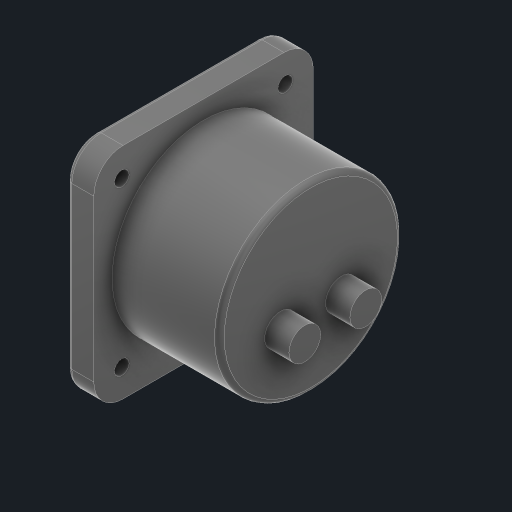
# Autodesk Inventor part: IIImeter
Saved by Autodesk Inventor 2024 (Build 280153000, 153)
## iProperties
Created: 2023-12-09
Part Number: IIImeter
Material: Acetal Resin, Black
Document SubType Name: Modeling
Designer: 16155
Density: 1.425 g/cm^3
Appearance: Smooth - Black
Author: 16155
Autodesk Inventor part; units mm, degrees
ref_plane "YZ Plane" through (0, 0, 0) normal (1, 0, 0) x (0, 1, 0)
ref_plane "XZ Plane" through (0, 0, 0) normal (0, 1, 0) x (-1, 0, 0)
ref_plane "XY Plane" through (0, 0, 0) normal (0, 0, 1) x (1, 0, 0)
sketch "Sketch1" plane through (0, 0, 0) normal (1, 0, 0) x (0, 1, 0)
  line L0 (-16.5, 22.5) -> (16.5, 22.5)
  line L1 (22.5, 16.5) -> (22.5, -16.5)
  line L2 (16.5, -22.5) -> (-16.5, -22.5)
  line L3 (-22.5, -16.5) -> (-22.5, 16.5)
  line L4 (-22.5, 22.5) -> (22.5, -22.5) construction
  line L5 (22.5, 22.5) -> (-22.5, -22.5) construction
  line L6 (-16.75, 16.75) -> (16.75, 16.75)
  line L7 (16.75, 16.75) -> (16.75, -16.75)
  line L8 (16.75, -16.75) -> (-16.75, -16.75)
  line L9 (-16.75, -16.75) -> (-16.75, 16.75)
  line L10 (-16.75, 16.75) -> (16.75, -16.75) construction
  line L11 (16.75, 16.75) -> (-16.75, -16.75) construction
  circle A0 centre (16.75, 16.75) radius 1.5
  circle A1 centre (-16.75, 16.75) radius 1.5
  circle A2 centre (-16.75, -16.75) radius 1.5
  circle A3 centre (16.75, -16.75) radius 1.5
  line L12 (4, 17.5) -> (-1, 17.5)
  line L13 (-4, 14.5) -> (-4, -14.5)
  line L14 (-1, -17.5) -> (4, -17.5)
  line L15 (4, -17.5) -> (4, 17.5)
  line L16 (4, 17.5) -> (-4, -17.5) construction
  line L17 (-4, 17.5) -> (4, -17.5) construction
  line L18 (22.5, 0) -> (17.32, 0)
  arc A4 (4, -17.5) -> (4, 17.5) centre (-0.8359, 0) ccw
  arc A5 (-1, 17.5) -> (-4, 14.5) centre (-1, 14.5) ccw
  arc A6 (-4, -14.5) -> (-1, -17.5) centre (-1, -14.5) ccw
  arc A7 (-16.5, 22.5) -> (-22.5, 16.5) centre (-16.5, 16.5) ccw
  arc A8 (-22.5, -16.5) -> (-16.5, -22.5) centre (-16.5, -16.5) ccw
  arc A9 (16.5, -22.5) -> (22.5, -16.5) centre (16.5, -16.5) ccw
  arc A10 (22.5, 16.5) -> (16.5, 22.5) centre (16.5, 16.5) ccw
  point P0 (0, 0)
  point P1 (6.1694, -16.75)
  point P2 (-2.9843, -16.75)
  point P3 (-2.9843, 16.75)
  point P4 (6.1694, 16.75)
  dimension "d0" = 45
  dimension "d1" = 45
  dimension "d2" = 33.5
  dimension "d3" = 33.5
  dimension "d4" = 3
  dimension "d7" = 360
  dimension "d9" = 35
  dimension "d10" = 8
  dimension "d11" = 5.18
  dimension "d12" = 3
  dimension "d13" = 6
  constraints: 38 end point, 15 point on circle, 12 point on line, 12 tangent, 11 centre point, 7 midpoint, 6 parallel, 4 equal radius, 4 horizontal, 3 perpendicular, 1 coincident, 9 other
  measures "d0" distance of L5.start L4.end
  measures "d1" distance of L4.end L5.end
  measures "d2" distance of L6.end L7.end
  measures "d3" distance of L7.end L8.end
  measures "d4" diameter of A0
  measures "d9" distance of L14.end L12.start
  measures "d10" distance of L16.end L14.end
  measures "d11" distance of L18.start L18.end
  measures "d12" radius of A5
  measures "d13" radius of A7
extrude "Extrusion1" add sketch "Sketch1" along normal blind 5.5 contours L0 A10 L1 A9 L2 A8 L3 A7 | L6 A5 L13 A6 L8 A2 L9 A1 | A5 L12 L15 L6 | L15 A4 L6 | L6 A0 L7 A4 | L15 L14 A6 L8 | L8 A4 L15 | A4 L7 A3 L8
sketch "Sketch2" plane through (5.5, 0, 0) normal (1, 0, 0) x (0, 0, -1)
  circle A0 centre (0, 0) radius 18.75
  dimension "d16" = 37.5
  constraints: 1 centre point, 1 coincident
  measures "d16" diameter of A0
extrude "Extrusion2" add sketch "Sketch2" along normal blind 22
fillet "Fillet1" radius 1 8 edges at (0, 20.7426, 20.7426) (0, 0, 22.5) (0, -20.7426, 20.7426) (0, -22.5, 0) (0, -20.7426, -20.7426) (0, 0, -22.5) (0, 20.7426, -20.7426) (0, 22.5, 0)
fillet "Fillet2" radius 1 6 edges at (0, 17.32, 0) (0, 1.5925, -16.75) (0, -4, 0) (0, -3.7343, 15.7343) (0, -3.7343, -15.7343) (0, 1.5925, 16.75)
sketch "Sketch3" plane through (27.5, 0, 0) normal (1, 0, 0) x (0, 0, -1)
  line L0 (-6.25, 4.3) -> (6.25, 4.3)
  line L1 (6.25, 4.3) -> (6.25, -4.3)
  line L2 (6.25, -4.3) -> (-6.25, -4.3)
  line L3 (-6.25, -4.3) -> (-6.25, 4.3)
  line L4 (-6.25, 4.3) -> (6.25, -4.3) construction
  line L5 (6.25, 4.3) -> (-6.25, -4.3) construction
  circle A0 centre (-6.25, -4.3) radius 3.25
  circle A1 centre (6.25, -4.3) radius 3.25
  point P0 (0, 0)
  dimension "d21" = 12.5
  dimension "d22" = 8.6
  dimension "d23" = 6.5
  dimension "d24" = 6.5
  constraints: 12 end point, 2 centre point, 2 midpoint, 2 parallel, 1 coincident, 1 horizontal, 1 perpendicular
  measures "d21" distance of L1.end L2.end
  measures "d22" distance of L0.end L1.end
  measures "d23" diameter of A0
  measures "d24" diameter of A1
extrude "Extrusion3" add sketch "Sketch3" along normal blind 5 contours A0 L2 L3 | L3 L2 A0 | A1 L2 L1 | L1 L2 A1
fillet "Fillet3" radius 1 1 edges at (27.5, 0, 18.75)
body "Solid1"
